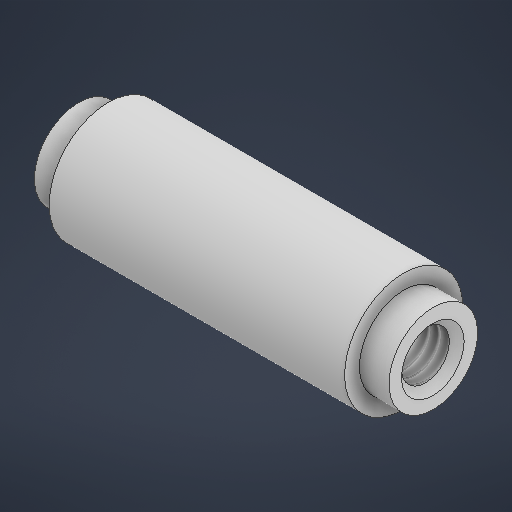
# Autodesk Inventor part: BaseSupport
Saved by Autodesk Inventor 2025.4 (Build 294407000, 407)
## iProperties
Created: 2026-05-26
Part Number: BaseSupport
Material: Generic
Document SubType Name: Modeling
Designer: VuQuan
Density: 1 g/cm^3
Appearance: Default
Author: VuQuan
Autodesk Inventor part; units mm, degrees
ref_plane "YZ Plane" through (0, 0, 0) normal (1, 0, 0) x (0, 1, 0)
ref_plane "XZ Plane" through (0, 0, 0) normal (0, 1, 0) x (-1, 0, 0)
ref_plane "XY Plane" through (0, 0, 0) normal (0, 0, 1) x (1, 0, 0)
sketch "Sketch1" plane through (0, 0, 0) normal (0, 0, 1) x (1, 0, 0)
  line L0 (-12, 0) -> (12, 0)
  line L1 (12, 0) -> (12, 3)
  line L2 (12, 3) -> (10, 3)
  line L3 (10, 3) -> (10, 4)
  line L4 (10, 4) -> (-10, 4)
  line L5 (-10, 4) -> (-10, 3)
  line L6 (-10, 3) -> (-12, 3)
  line L7 (-12, 3) -> (-12, 0)
  point P0 (0, 0)
  point P1 (0, 0)
  dimension "d0" = 24
  dimension "d1" = 6
  dimension "d2" = 8
  dimension "d3" = 2
  constraints: 16 end point, 6 perpendicular, 2 collinear, 1 coincident, 1 horizontal, 1 midpoint
  measures "d0" distance of L0.start L0.end
  measures "d1" diameter of L6 L0
  measures "d2" diameter of L4 L0
  measures "d3" distance between parallel lines of L7 L5
revolve "Revolution1" add sketch "Sketch1" angle 360 about axis through (-12, 0, 0) along (1, 0, 0)
sketch "Sketch2" plane through (12, 0, 0) normal (1, 0, 0) x (0, 0, -1)
  point P0 (0, 0)
  point P1 (-0.1005, -0.6753)
  point P2 (-0.0327, -0.0508)
hole "Hole1" at (12, -0.0508, 0.0327) direction (-1, 0, 0) diameter 3.242 end up to face face through (-12, 0.5681, -0.823) facing (-1, 0, 0) thread size "M4x0.7" class "6H" standard "ISO Metric profile"
chamfer "Chamfer1" distance 0.5 angle 45 2 edges at (12, -0.0508, 1.6537) (-12, -0.0508, 1.6537)
body "Solid1"
